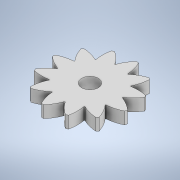
# Autodesk Inventor part: bánh răng 1
Saved by Autodesk Inventor 2020 (Build 240168000, 168)
## iProperties
Created: 2022-11-27
Part Number: bánh răng 1
Material: Generic
Document SubType Name: Modeling
Designer: ADMIN
Density: 1 g/cm^3
Appearance: Default
Author: ADMIN
Autodesk Inventor part; units mm, degrees
ref_plane "YZ Plane" through (0, 0, 0) normal (1, 0, 0) x (0, 1, 0)
ref_plane "XZ Plane" through (0, 0, 0) normal (0, 1, 0) x (-1, 0, 0)
ref_plane "XY Plane" through (0, 0, 0) normal (0, 0, 1) x (1, 0, 0)
sketch "Sketch5" plane through (0, 0, 0) normal (0, 1, 0) x (-1, 0, 0)
  line L0 (0, 0) -> (0, -7.7608)
  arc A0 (-2.2486, -13.8182) -> (-1.5122, -13.9181) centre (0, 0) ccw
  arc A1 (-1.5122, -13.9181) -> (-0.5252, -12.7176) centre (-10.3455, -5.6492) ccw
  arc A2 (-1.5122, -13.9181) -> (1.0504, -9.7156) centre (-10.3455, -5.6492) ccw
  arc A3 (-3.5996, -9.0851) -> (-2.2486, -13.8182) centre (8.4677, -8.2001) ccw
  arc A4 (1.4452, -9.3894) -> (1.0504, -9.7156) centre (1.5213, -9.8836) ccw
  arc A5 (-3.5996, -9.0851) -> (-3.8933, -8.6656) centre (-4.0982, -9.1217) ccw
  line L1 (0, 0) -> (1.4452, -9.3894)
  line L2 (0, 0) -> (-3.8933, -8.6656)
  point P0 (-0.5252, -12.7176)
  dimension "d50" = 28
  dimension "d53" = 0.5
  constraints: 12 point on circle, 6 centre point, 6 end point, 3 coincident, 2 tangent, 1 equal radius, 1 vertical
  measures "d50" diameter of A0
  measures "d53" radius of A4
extrude "Extrusion4" add sketch "Sketch5" along normal blind 4
pattern_circular "Circular Pattern1" count 12 over 360 about axis through (0, 0, 0) along (0, 1, 0) of "Extrusion4"
sketch "Sketch6" plane through (0, 4, 0) normal (0, 1, 0) x (1, 0, 0)
  circle A0 centre (0, 0) radius 2.75
  dimension "d59" = 5.5
  constraints: 1 centre point, 1 coincident
  measures "d59" diameter of A0
extrude "Extrusion5" cut sketch "Sketch6" against normal blind 4
body "Solid3"
